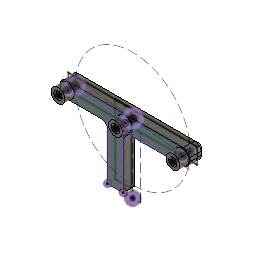
ThymioPipeLeft (Autodesk Fusion 360 design; units mm, degrees)
part number: 2026-07-25-13-46-56-369
Autodesk Fusion 360 part; units mm, degrees
sketch "Sketch1" plane through (0, 0, 0) normal (0, 1, 0) x (1, 0, 0)
  line L0 (0, 0) -> (0, -36) construction
  line L1 (0, -36) -> (-30, -36)
  line L2 (0, -36) -> (30, -36)
  line L3 (-4.1, 0) -> (4.1, 0) construction
  line L4 (4.1, 0) -> (4.1, -40.2) construction
  line L5 (4.1, -40.2) -> (-4.1, -40.2) construction
  line L6 (-4.1, -40.2) -> (-4.1, 0) construction
  line L7 (-33.625, -40.1) -> (33.625, -40.1)
  line L8 (33.625, -40.1) -> (33.625, -31.9)
  line L9 (33.625, -31.9) -> (-33.625, -31.9)
  line L10 (-33.625, -31.9) -> (-33.625, -40.1)
  circle A0 centre (0, -36) radius 30 construction
  line L11 (-33.625, -40.1) -> (33.625, -31.9) construction
  line L12 (-9.1, -40.1) -> (-0.9, -40.1)
  line L13 (-0.9, -40.1) -> (-0.9, -4.1)
  line L14 (-0.9, -4.1) -> (-9.1, -4.1)
  line L15 (-9.1, -4.1) -> (-9.1, -40.1)
  line L16 (-5, -4.1) -> (-5, -36)
  point P0 (0, -36)
  dimension "d9" = 36
  dimension "d10" = 30
  dimension "d11" = 30
  dimension "d12" = 8.2
  dimension "d13" = 40.2
  dimension "d14" = 67.25
  dimension "d15" = 8.2
  dimension "d52" = 8.2
  dimension "d53" = 36
  dimension "d54" = 35
  constraint coincident L0.start origin
  constraint vertical L0
  constraint perpendicular L0 L1
  constraint perpendicular L0 L2
  constraint horizontal L3
  constraint vertical L4
  constraint horizontal L5
  constraint vertical L6
  constraint midpoint L0.start L3
  constraint horizontal L7
  constraint vertical L8
  constraint horizontal L9
  constraint vertical L10
  constraint coincident L2.end A0
  constraint coincident L1.end A0
  constraint coincident L11 P0
  constraint midpoint L11 P0
  constraint coincident P0 L0.end
  constraint coincident L1 P0
  constraint horizontal L12
  constraint vertical L13
  constraint horizontal L14
  constraint vertical L15
  constraint coincident L7 L12.start
  constraint midpoint L14 L16.start
  constraint coincident L1 L16.end
  constraint perpendicular L1 L16
  measures "d9" distance of L0.start P0
  measures "d10" distance of P0 L1.end
  measures "d11" distance of P0 L2.end
  measures "d12" distance of L3.start L3.end
  measures "d13" distance of L3.start L5.end
  measures "d14" distance of L7.start L7.end
  measures "d15" distance of L7.start L9.end
  measures "d52" distance of L13.end L14.end
  measures "d53" distance of L12.start L14.end
  measures "d54" distance of L2.end L16
extrude "Extrude1" add sketch "Sketch1" along normal mid plane 8.2
ref_plane "WorkPlane1" through (0, 0, 36) normal (0, 0, 1) x (1, 0, 0)
sketch "Sketch2" plane through (0, 0, 36) normal (0, 0, 1) x (1, 0, 0)
  line L0 (30, 0) -> (30, -9)
  line L1 (0, 0) -> (0, -9)
  line L2 (-30, 0) -> (-30, -9)
  line L3 (0, 0) -> (-30, 0)
  point P0 (-30, 0)
  point P1 (30, 0)
  dimension "d20" = 9
  dimension "d21" = 9
  dimension "d22" = 9
  constraint vertical L0
  constraint vertical L1
  constraint vertical L2
  constraint coincident L0.start P1
  constraint coincident L1.start L3.start
  constraint coincident P0 L3
  constraint coincident P0 L2.start
  measures "d20" distance of L0.start L0.end
  measures "d21" distance of L1.start L1.end
  measures "d22" distance of P0 L2.end
sketch "Sketch3" plane through (0, -4.1, 0) normal (0, -1, 0) x (1, 0, 0)
  line L0 (-33.625, 31.9) -> (-9.1, 31.9)
  line L1 (33.625, 31.9) -> (33.625, 40.1)
  line L2 (33.625, 40.1) -> (-33.625, 40.1)
  line L3 (-33.625, 40.1) -> (-33.625, 31.9)
  circle A0 centre (-30, 36) radius 3.625
  circle A1 centre (0, 36) radius 3.625
  circle A2 centre (30, 36) radius 3.625
  line L4 (-9.1, 31.9) -> (-9.1, 4.1)
  line L5 (-9.1, 4.1) -> (-0.9, 4.1)
  line L6 (-0.9, 4.1) -> (-0.9, 31.9)
  line L7 (-0.9, 31.9) -> (33.625, 31.9)
  point P0 (30, 36)
  point P1 (0, 36)
  point P2 (-30, 36)
  dimension "d23" = 7.25
  dimension "d24" = 7.25
  dimension "d25" = 7.25
  constraint coincident P0 A2.centre
  constraint coincident P1 A1.centre
  constraint coincident P2 A0.centre
  measures "d23" diameter of A0
  measures "d24" diameter of A1
  measures "d25" diameter of A2
extrude "Extrude2" add sketch "Sketch3" along normal blind 4.9 contours A2 | A0 | A1
pipe "Pipe5" cut diameter 4.2 path "Sketch1" along L16
pipe "Pipe6" cut diameter 4.2 path "Sketch1" along L1 L2
pipe "Pipe7" cut diameter 3.25 path "Sketch2" along L2 L3
pipe "Pipe8" cut diameter 3.25 path "Sketch2" along L1
pipe "Pipe9" cut diameter 3.25 path "Sketch2" along L0
fillet "Fillet3" offset 0.5 second offset 1 3 edges at (28.485, -9, 36.5876) (-1.515, -9, 36.5876) (-28.485, -9, 35.4124) measured on face at (32.9433, -9, 35.7794) measured on face at (2.9388, -9, 35.7392) measured on face at (-27.0567, -9, 36.2206)
fillet "Fillet4" offset 3.25 second offset 3 6 edges at (-33.625, 0, 40.1) (-33.625, 0, 31.9) (-9.1, 0, 31.9) (-0.9, 0, 31.9) (33.625, 0, 31.9) (33.625, 0, 40.1) measured on face at (-33.625, 1.3667, 36) measured on face at (-17.275, 1.3667, 31.9) measured on face at (-9.1, 1.3667, 13.3667) measured on face at (22.1167, 1.3667, 31.9) measured on face at (33.625, 1.3667, 36) measured on face at (11.2083, -1.3667, 40.1)
sketch "Sketch4" plane through (0, 4.1, 0) normal (0, 1, 0) x (-1, 0, 0)
  spline S0 degree 3 poles (-33.5, 37.1) (-33.5, 37.4961) (-33.4215, 37.8883) (-33.1149, 38.6241) (-32.8881, 38.9595) (-32.327, 39.5105) (-32.0025, 39.7251) (-31.2828, 40.0227) (-30.8933, 40.1) (-30.5, 40.1) knots 0 0 0 0 0.118836 0.118836 0.239117 0.239117 0.354753 0.354753 0.472749 0.472749 0.472749 0.472749
  line L0 (-33.5, 37.1) -> (-33.5, 34.9)
  spline S1 degree 3 poles (-30.5, 31.9) (-30.8961, 31.9) (-31.2883, 31.9785) (-32.0241, 32.2851) (-32.3595, 32.5119) (-32.9105, 33.073) (-33.1251, 33.3975) (-33.4227, 34.1172) (-33.5, 34.5067) (-33.5, 34.9) knots 0 0 0 0 0.118836 0.118836 0.239117 0.239117 0.354753 0.354753 0.472749 0.472749 0.472749 0.472749
  line L1 (-30.5, 31.9) -> (-2.1, 31.9)
  spline S2 degree 3 poles (0.9, 28.9) (0.9, 29.2961) (0.8215, 29.6883) (0.5149, 30.4241) (0.2881, 30.7595) (-0.273, 31.3105) (-0.5975, 31.5251) (-1.3172, 31.8227) (-1.7067, 31.9) (-2.1, 31.9) knots 0 0 0 0 0.118836 0.118836 0.239117 0.239117 0.354753 0.354753 0.472749 0.472749 0.472749 0.472749
  line L2 (0.9, 28.9) -> (0.9, 4.1)
  line L3 (0.9, 4.1) -> (9.1, 4.1)
  line L4 (9.1, 4.1) -> (9.1, 28.9)
  spline S3 degree 3 poles (12.1, 31.9) (11.7039, 31.9) (11.3117, 31.8215) (10.5759, 31.5149) (10.2405, 31.2881) (9.6895, 30.727) (9.4749, 30.4025) (9.1773, 29.6828) (9.1, 29.2933) (9.1, 28.9) knots 0 0 0 0 0.118836 0.118836 0.239117 0.239117 0.354753 0.354753 0.472749 0.472749 0.472749 0.472749
  spline S4 degree 3 poles (33.5, 34.9) (33.5, 34.5039) (33.4215, 34.1117) (33.1149, 33.3759) (32.8881, 33.0405) (32.327, 32.4895) (32.0025, 32.2749) (31.2828, 31.9773) (30.8933, 31.9) (30.5, 31.9) knots 0 0 0 0 0.118836 0.118836 0.239117 0.239117 0.354753 0.354753 0.472749 0.472749 0.472749 0.472749
  line L5 (33.5, 34.9) -> (33.5, 37.1)
  spline S5 degree 3 poles (30.5, 40.1) (30.8961, 40.1) (31.2883, 40.0215) (32.0241, 39.7149) (32.3595, 39.4881) (32.9105, 38.927) (33.1251, 38.6025) (33.4227, 37.8828) (33.5, 37.4933) (33.5, 37.1) knots 0 0 0 0 0.118836 0.118836 0.239117 0.239117 0.354753 0.354753 0.472749 0.472749 0.472749 0.472749
  line L6 (30.5, 40.1) -> (-30.5, 40.1)
  line L7 (-25.5806, 32.6021) -> (61.8548, 32.6021) construction
  line L8 (61.8548, 32.6021) -> (61.8548, 40.7394) construction
  line L9 (61.8548, 40.7394) -> (-25.5806, 40.7394) construction
  line L10 (-25.5806, 40.7394) -> (-25.5806, 32.6021) construction
  line L11 (12.1, 31.9) -> (30.5, 31.9)
  dimension "d81" = 6
  dimension "d82" = 0
extrude "Extrude3" [suppressed]
fillet "Fillet5" offset 0.5 second offset 1 1 edges at (-6.9579, -0.7594, 4.1) measured on face at (-5.0523, 3.4314, 4.1)
extrude "Extrude4" [suppressed]
chamfer "Chamfer1" distance 2 angle 45 13 edges at (33.625, 4.1, 36.125) (32.7847, 4.1, 32.8942) (16.4875, 4.1, 31.9) (0.0942, 4.1, 31.0597) (-0.9, 4.1, 16.5) (-9.1, 4.1, 16.375) (-9.9403, 4.1, 30.9058) (-21.2375, 4.1, 31.9) (-32.6308, 4.1, 32.7403) (-33.625, 4.1, 35.875) (-32.7847, 4.1, 39.1058) (-0.125, 4.1, 40.1) (32.6308, 4.1, 39.2597) tangent chain off
equation "WallThickness = 2 mm"
equation "PumpHoleDiameter = 4.2 mm"
equation "SizeKOffset = 5.5 mm"
equation "ValveHoleDiameter = 3.25 mm"
equation "SizeE = 34 mm + 2 mm"
equation "SizeF = 30 mm"
equation "SizeG = 30 mm"
equation "SizeH = 7 mm + 2 mm"
equation "d9 = SizeE"
equation "d10 = SizeF"
equation "d11 = SizeG"
equation "d12 = PumpHoleDiameter + 2 * WallThickness"
equation "d13 = SizeE + PumpHoleDiameter"
equation "d14 = SizeF + SizeG + 2 * WallThickness + ValveHoleDiameter"
equation "d15 = PumpHoleDiameter + 2 * WallThickness"
equation "d16 = ( PumpHoleDiameter + 2 * WallThickness ) / 2"
equation "d18 = SizeE"
equation "d20 = SizeH"
equation "d21 = SizeH"
equation "d22 = SizeH"
equation "d23 = ValveHoleDiameter + 2 * WallThickness"
equation "d24 = ValveHoleDiameter + 2 * WallThickness"
equation "d25 = ValveHoleDiameter + 2 * WallThickness"
equation "d26 = SizeH - ( PumpHoleDiameter / 2 ) - WallThickness"
equation "d52 = PumpHoleDiameter + 2 * WallThickness"
equation "d53 = SizeE"
equation "d57 = PumpHoleDiameter"
equation "d61 = PumpHoleDiameter"
equation "d65 = ValveHoleDiameter"
equation "d69 = ValveHoleDiameter"
equation "d73 = ValveHoleDiameter"
equation "d79 = min(ValveHoleDiameter; PumpHoleDiameter)"
equation "d82 = 'v2'"
